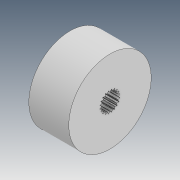
# Autodesk Inventor part: roda certa
Saved by Autodesk Inventor 2021 (Build 250183000, 183)
## iProperties
Created: 2020-10-21
Part Number: roda certa
Material: Genérico
Document SubType Name: Modeling
Designer: evert
Density: 1 g/cm^3
Appearance: Padrão
Author: evert
Autodesk Inventor part; units mm, degrees
ref_plane "YZ Plane" through (0, 0, 0) normal (1, 0, 0) x (0, 1, 0)
ref_plane "XZ Plane" through (0, 0, 0) normal (0, 1, 0) x (-1, 0, 0)
ref_plane "XY Plane" through (0, 0, 0) normal (0, 0, 1) x (1, 0, 0)
sketch "Esboço2" plane through (0, 0, 0) normal (0, 0, 1) x (1, 0, 0)
  line L0 (0, 0) -> (9.5, 0)
  line L1 (9.5, 0) -> (9.5, 9.8)
  line L2 (9.5, 9.8) -> (0, 9.8)
  line L3 (0, 9.8) -> (0, 0)
  dimension "d0" = 9.5
  dimension "d1" = 9.8
  constraints: 8 end point, 2 parallel, 1 horizontal, 1 perpendicular
  measures "d0" distance of L1.end L2.end
  measures "d1" distance of L0.end L1.end
revolve "Revolução1" add sketch "Esboço2" angle 360 about axis through (0, 0, 0) along (1, 0, 0)
sketch "Esboço3" plane through (0, 0, 0) normal (-1, 0, 0) x (0, 0, 1)
  circle A0 centre (0, 0) radius 1.75
  dimension "d3" = 3.5
  constraints: 1 centre point, 1 coincident
  measures "d3" diameter of A0
extrude "Extrusão1" cut sketch "Esboço3" against normal blind 4.85
sketch "Esboço4" plane through (0, 0, 0) normal (-1, 0, 0) x (0, 0, 1)
  circle A0 centre (0, 0) radius 4.5
  dimension "d6" = 9
  constraints: 1 centre point, 1 coincident
  measures "d6" diameter of A0
extrude "Extrusão2" cut sketch "Esboço4" against normal blind 2
sketch "Esboço8" plane through (9.5, 0, 0) normal (1, 0, 0) x (0, 0, -1)
  circle A0 centre (0, 0) radius 2
  circle A1 centre (0, 0) radius 2.4
  line L0 (2, 0) -> (2, 0.05)
  line L1 (2, 0) -> (1.9994, -0.05)
  line L2 (1.9994, -0.05) -> (2, 0.05)
  line L3 (2, 0.05) -> (2.3777, 0.3266)
  line L4 (1.9994, -0.05) -> (2.3779, -0.3252)
  arc A2 (2.3779, -0.3252) -> (2.3777, 0.3266) centre (0, 0) ccw
  line L5 (2.3777, 0.3266) -> (2.3777, 0.3266)
  line L6 (2.3777, 0.3266) -> (2.3777, 0.3266)
  line L7 (2.3777, 0.3266) -> (2.3777, 0.3266)
  line L8 (2.3779, -0.3252) -> (2.3706, -0.3747)
  line L9 (2.3706, -0.3747) -> (2.3779, -0.3252)
  line L10 (2.3777, 0.3266) -> (2.3777, 0.3266)
  line L11 (2.3777, 0.3266) -> (2.3777, 0.3266)
  line L12 (1.8867, 0.6656) -> (2.1604, 1.0453)
  line L13 (1.917, 0.5703) -> (1.8867, 0.6656)
  line L14 (1.917, 0.5703) -> (2.362, 0.4255)
  line L15 (2.3703, 0.3762) -> (2.362, 0.4255)
  arc A3 (2.362, 0.4255) -> (2.1604, 1.0453) centre (0, 0) ccw
  line L16 (1.5886, 1.216) -> (1.7316, 1.6618)
  line L17 (1.6469, 1.1348) -> (1.5886, 1.216)
  line L18 (1.6469, 1.1348) -> (2.1149, 1.1346)
  line L19 (2.1381, 1.0903) -> (2.1149, 1.1346)
  arc A4 (2.1149, 1.1346) -> (1.7316, 1.6618) centre (0, 0) ccw
  line L20 (1.1351, 1.6474) -> (1.1334, 2.1155)
  line L21 (1.2157, 1.5881) -> (1.1351, 1.6474)
  line L22 (1.2157, 1.5881) -> (1.6608, 1.7326)
  line L23 (1.6965, 1.6976) -> (1.6608, 1.7326)
  arc A5 (1.6608, 1.7326) -> (1.1334, 2.1155) centre (0, 0) ccw
  line L24 (0.5705, 1.9176) -> (0.4241, 2.3622)
  line L25 (0.6654, 1.8861) -> (0.5705, 1.9176)
  line L26 (0.6654, 1.8861) -> (1.0441, 2.161)
  line L27 (1.0889, 2.1388) -> (1.0441, 2.161)
  arc A6 (1.0441, 2.161) -> (0.4241, 2.3622) centre (0, 0) ccw
  line L28 (-0.05, 2) -> (-0.3266, 2.3777)
  line L29 (0.05, 1.9994) -> (-0.05, 2)
  line L30 (0.05, 1.9994) -> (0.3252, 2.3779)
  line L31 (0.3747, 2.3706) -> (0.3252, 2.3779)
  arc A7 (0.3252, 2.3779) -> (-0.3266, 2.3777) centre (0, 0) ccw
  line L32 (-0.6656, 1.8867) -> (-1.0453, 2.1604)
  line L33 (-0.5703, 1.917) -> (-0.6656, 1.8867)
  line L34 (-0.5703, 1.917) -> (-0.4255, 2.362)
  line L35 (-0.3762, 2.3703) -> (-0.4255, 2.362)
  arc A8 (-0.4255, 2.362) -> (-1.0453, 2.1604) centre (0, 0) ccw
  line L36 (-1.216, 1.5886) -> (-1.6618, 1.7316)
  line L37 (-1.1348, 1.6469) -> (-1.216, 1.5886)
  line L38 (-1.1348, 1.6469) -> (-1.1346, 2.1149)
  line L39 (-1.0903, 2.1381) -> (-1.1346, 2.1149)
  arc A9 (-1.1346, 2.1149) -> (-1.6618, 1.7316) centre (0, 0) ccw
  line L40 (-1.6474, 1.1351) -> (-2.1155, 1.1334)
  line L41 (-1.5881, 1.2157) -> (-1.6474, 1.1351)
  line L42 (-1.5881, 1.2157) -> (-1.7326, 1.6608)
  line L43 (-1.6976, 1.6965) -> (-1.7326, 1.6608)
  arc A10 (-1.7326, 1.6608) -> (-2.1155, 1.1334) centre (0, 0) ccw
  line L44 (-1.9176, 0.5705) -> (-2.3622, 0.4241)
  line L45 (-1.8861, 0.6654) -> (-1.9176, 0.5705)
  line L46 (-1.8861, 0.6654) -> (-2.161, 1.0441)
  line L47 (-2.1388, 1.0889) -> (-2.161, 1.0441)
  arc A11 (-2.161, 1.0441) -> (-2.3622, 0.4241) centre (0, 0) ccw
  line L48 (-2, -0.05) -> (-2.3777, -0.3266)
  line L49 (-1.9994, 0.05) -> (-2, -0.05)
  line L50 (-1.9994, 0.05) -> (-2.3779, 0.3252)
  line L51 (-2.3706, 0.3747) -> (-2.3779, 0.3252)
  arc A12 (-2.3779, 0.3252) -> (-2.3777, -0.3266) centre (0, 0) ccw
  line L52 (-1.8867, -0.6656) -> (-2.1604, -1.0453)
  line L53 (-1.917, -0.5703) -> (-1.8867, -0.6656)
  line L54 (-1.917, -0.5703) -> (-2.362, -0.4255)
  line L55 (-2.3703, -0.3762) -> (-2.362, -0.4255)
  arc A13 (-2.362, -0.4255) -> (-2.1604, -1.0453) centre (0, 0) ccw
  line L56 (-1.5886, -1.216) -> (-1.7316, -1.6618)
  line L57 (-1.6469, -1.1348) -> (-1.5886, -1.216)
  line L58 (-1.6469, -1.1348) -> (-2.1149, -1.1346)
  line L59 (-2.1381, -1.0903) -> (-2.1149, -1.1346)
  arc A14 (-2.1149, -1.1346) -> (-1.7316, -1.6618) centre (0, 0) ccw
  line L60 (-1.1351, -1.6474) -> (-1.1334, -2.1155)
  line L61 (-1.2157, -1.5881) -> (-1.1351, -1.6474)
  line L62 (-1.2157, -1.5881) -> (-1.6608, -1.7326)
  line L63 (-1.6965, -1.6976) -> (-1.6608, -1.7326)
  arc A15 (-1.6608, -1.7326) -> (-1.1334, -2.1155) centre (0, 0) ccw
  line L64 (-0.5705, -1.9176) -> (-0.4241, -2.3622)
  line L65 (-0.6654, -1.8861) -> (-0.5705, -1.9176)
  line L66 (-0.6654, -1.8861) -> (-1.0441, -2.161)
  line L67 (-1.0889, -2.1388) -> (-1.0441, -2.161)
  arc A16 (-1.0441, -2.161) -> (-0.4241, -2.3622) centre (0, 0) ccw
  line L68 (0.05, -2) -> (0.3266, -2.3777)
  line L69 (-0.05, -1.9994) -> (0.05, -2)
  line L70 (-0.05, -1.9994) -> (-0.3252, -2.3779)
  line L71 (-0.3747, -2.3706) -> (-0.3252, -2.3779)
  arc A17 (-0.3252, -2.3779) -> (0.3266, -2.3777) centre (0, 0) ccw
  line L72 (0.6656, -1.8867) -> (1.0453, -2.1604)
  line L73 (0.5703, -1.917) -> (0.6656, -1.8867)
  line L74 (0.5703, -1.917) -> (0.4255, -2.362)
  line L75 (0.3762, -2.3703) -> (0.4255, -2.362)
  arc A18 (0.4255, -2.362) -> (1.0453, -2.1604) centre (0, 0) ccw
  line L76 (1.216, -1.5886) -> (1.6618, -1.7316)
  line L77 (1.1348, -1.6469) -> (1.216, -1.5886)
  line L78 (1.1348, -1.6469) -> (1.1346, -2.1149)
  line L79 (1.0903, -2.1381) -> (1.1346, -2.1149)
  arc A19 (1.1346, -2.1149) -> (1.6618, -1.7316) centre (0, 0) ccw
  line L80 (1.6474, -1.1351) -> (2.1155, -1.1334)
  line L81 (1.5881, -1.2157) -> (1.6474, -1.1351)
  line L82 (1.5881, -1.2157) -> (1.7326, -1.6608)
  line L83 (1.6976, -1.6965) -> (1.7326, -1.6608)
  arc A20 (1.7326, -1.6608) -> (2.1155, -1.1334) centre (0, 0) ccw
  line L84 (1.9176, -0.5705) -> (2.3622, -0.4241)
  line L85 (1.8861, -0.6654) -> (1.9176, -0.5705)
  line L86 (1.8861, -0.6654) -> (2.161, -1.0441)
  line L87 (2.1388, -1.0889) -> (2.161, -1.0441)
  arc A21 (2.161, -1.0441) -> (2.3622, -0.4241) centre (0, 0) ccw
  point P0 (1.9998, 0.025)
  point P1 (1.8942, 0.6418)
  point P2 (1.6032, 1.1957)
  point P3 (1.1553, 1.6326)
  point P4 (0.5942, 1.9097)
  point P5 (-0.025, 1.9998)
  point P6 (-0.6418, 1.8942)
  point P7 (-1.1957, 1.6032)
  point P8 (-1.6326, 1.1553)
  point P9 (-1.9097, 0.5942)
  point P10 (-1.9998, -0.025)
  point P11 (-1.8942, -0.6418)
  point P12 (-1.6032, -1.1957)
  point P13 (-1.1553, -1.6326)
  point P14 (-0.5942, -1.9097)
  point P15 (0.025, -1.9998)
  point P16 (0.6418, -1.8942)
  point P17 (1.1957, -1.6032)
  point P18 (1.6326, -1.1553)
  point P19 (1.9097, -0.5942)
  dimension "d35" = 4
  dimension "d36" = 4.8
  dimension "d37" = 0.05
  dimension "d38" = 0.05
  dimension "d39" = 0.05
  dimension "d44" = 360
  constraints: 176 end point, 40 point on circle, 20 centre point, 2 coincident, 2 vertical, 1 collinear, 241 other
  measures "d37" distance of L0.start L0.end
  measures "d38" distance of L0.start L1.end
  measures "d39" distance of L4.end L8.end
extrude "Extrusão3" cut sketch "Esboço8" against normal blind 3.5 contours A0 | A0 L14 A1 L3 | L4 A1 L84 A0 | A0 L18 A1 L12 | L86 A1 L80 A0 | A0 L22 A1 L16 | L82 A1 L76 A0 | A0 L26 A1 L20 | L78 A1 L72 A0 | A0 L30 A1 L24 | L74 A1 L68 A0 | A0 L34 A1 L28 | L70 A1 L64 A0 | A0 L38 A1 L32 | L66 A1 L60 A0 | A0 L42 A1 L36 | L62 A1 L56 A0 | A0 L46 A1 L40 | L58 A1 L52 A0 | A0 L50 A1 L44 | L54 A1 L48 A0
